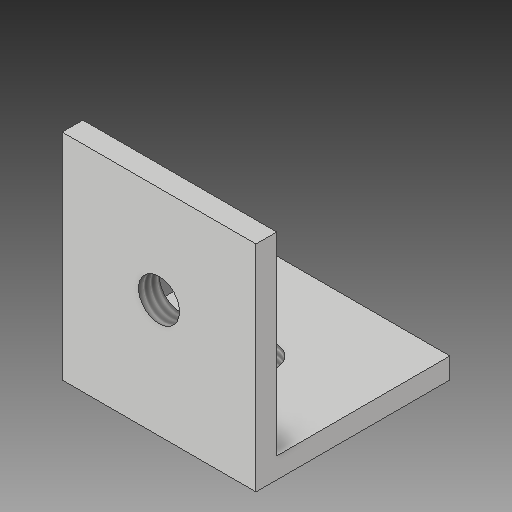
# Autodesk Inventor part: Esquinero
Saved by Autodesk Inventor 2019 (Build 230136000, 136)
## iProperties
Created: 2019-11-21
Part Number: Esquinero
Material: Generic
Document SubType Name: Modeling
Designer: felix
Density: 1 g/cm^3
Appearance: Default
Mass: 4.53902 g
Surface Area: 36.4154 cm^2
Volume: 4.53902 cm^3
Author: felix
Autodesk Inventor part; units mm, degrees
ref_plane "YZ Plane" through (0, 0, 0) normal (1, 0, 0) x (0, 1, 0)
ref_plane "XZ Plane" through (0, 0, 0) normal (0, 1, 0) x (-1, 0, 0)
ref_plane "XY Plane" through (0, 0, 0) normal (0, 0, 1) x (1, 0, 0)
sketch "Sketch1" plane through (0, 0, 0) normal (0, 0, 1) x (1, 0, 0)
  line L0 (-28, 28) -> (0, 28)
  line L1 (0, 28) -> (0, 0)
  line L2 (0, 0) -> (-28, 0)
  line L3 (-28, 0) -> (-28, 28)
  dimension "d0" = 28
  dimension "d1" = 28
  constraints: 8 end point, 2 parallel, 1 coincident, 1 horizontal, 1 perpendicular
  measures "d0" distance of L0.start L0.end
  measures "d1" distance of L2.end L0.start
extrude "Extrusion1" add sketch "Sketch1" along normal blind 3
sketch "Sketch2" plane through (0, 0, 3) normal (0, 0, 1) x (1, 0, 0)
  line L0 (0, 28) -> (-28, 28) projected
  line L1 (0, 0) -> (0, 28) projected
  point P0 (-14, 14)
  dimension "d4" = 14
  dimension "d5" = 14
  measures "d4" distance from line of L0 point (-14, 14)
  measures "d5" distance from line of L1 point (-14, 14)
hole "Hole1" at (-14, 14, 3) direction (0, 0, -1) diameter 5.917 depth 19.1 tip angle 118 thread size "M7x1" class "6H" standard "ANSI Metric M Profile"
sketch "Sketch3" plane through (0, 0, 3) normal (0, 0, 1) x (1, 0, 0)
  line L0 (-28, 0) -> (0, 0) projected
  line L1 (0, 0) -> (-28, 0)
  line L2 (-28, 0) -> (-28, -3)
  line L3 (-28, -3) -> (0, -3)
  line L4 (0, -3) -> (0, 0)
  line L5 (-28, 28) -> (-28, 0) projected
  dimension "d13" = 3
  constraints: 8 end point, 2 parallel, 1 horizontal, 1 perpendicular, 1 point on line
  measures "d13" distance of L2.end L1.end
extrude "Extrusion2" add sketch "Sketch3" against normal blind 28
sketch "Sketch4" plane through (-28, -3, 3) normal (0, -1, 0) x (1, 0, 0)
  line L0 (0, 0) -> (28, 0) projected
  line L1 (28, 0) -> (28, -28) projected
  point P0 (28, -3)
  point P1 (14, -14)
  dimension "d16" = 14
  dimension "d17" = 14
  measures "d16" distance from line of L0 point (14, -14)
  measures "d17" distance from line of L1 point (14, -14)
hole "Hole2" at (-14, -3, -11) direction (0, 1, 0) diameter 5.917 depth 19.1 tip angle 118 thread size "M7x1" class "6H" standard "ANSI Metric M Profile"
body "Solid1"
